connector_single_magnet (Autodesk Fusion 360 design; units mm, degrees)
Autodesk Fusion 360 part; units mm, degrees
sketch "Sketch1" plane through (0, 0, 0) normal (0, 1, 0) x (1, 0, 0)
  line L0 (0, 0) -> (-34, 0)
  line L1 (-34, 0) -> (-34, -10)
  line L2 (-34, -10) -> (0, -10)
  line L3 (0, -10) -> (0, 0)
  line L4 (0, -5) -> (-34, -5) construction
  circle A0 centre (-17, -5) radius 4
  circle A1 centre (-30, -5) radius 2
  line L5 (-17, -2.5) -> (0, -2.5) construction
  line L6 (-17, -5) -> (-17, 0) construction
  line L7 (-17, -5) -> (-17, -10) construction
  line L8 (-22, -5) -> (-27, -5)
  arc A2 (-22, -5) -> (-27, -5) centre (-24.5, -5) ccw
  arc A3 (-27, -5) -> (-22, -5) centre (-24.5, -5) ccw
  line L9 (-7, -5) -> (-12, -5)
  arc A4 (-7, -5) -> (-12, -5) centre (-9.5, -5) ccw
  arc A5 (-12, -5) -> (-7, -5) centre (-9.5, -5) ccw
  line L10 (-9.5, -5) -> (-9.5, -10) construction
  line L11 (-9.5, -5) -> (-9.5, 0) construction
  line L12 (-30, -5) -> (-30, -10) construction
  line L13 (-30, -5) -> (-30, 0) construction
  circle A6 centre (-9.5, -5) radius 3.5
  circle A7 centre (-17, -5) radius 5
  circle A8 centre (-24.5, -5) radius 3.5
  circle A9 centre (-30, -5) radius 3
  line L14 (-8.8, -1.5707) -> (-16, -0.101)
  line L15 (-8.8, -8.4293) -> (-16, -9.899)
  line L16 (-25.2, -8.4293) -> (-18, -9.899)
  line L17 (-18, -0.101) -> (-25.2, -1.5707)
  line L18 (-24.8182, -1.5145) -> (-30.2727, -2.0124)
  line L19 (-24.8182, -8.4855) -> (-30.2727, -7.9876)
  dimension "d2" = 8
  dimension "d3" = 10
  dimension "d4" = 5
  dimension "d5" = 5
  dimension "d6" = 7.5
  dimension "d7" = 7.5
  dimension "d8" = 5.5
  dimension "d9" = 4
  dimension "d12" = 4
  dimension "d41" = 6
  dimension "d42" = 7
  dimension "d43" = 10
  dimension "d44" = 7
  constraint horizontal L0
  constraint vertical L1
  constraint horizontal L2
  constraint vertical L3
  constraint coincident L0.start L3.end
  constraint midpoint L3 L4.start
  constraint midpoint L1 L4.end
  constraint midpoint L4 A0.centre
  constraint coincident L4 A4.centre
  constraint coincident L3 L5.end
  constraint perpendicular L3 L5
  constraint coincident A0.centre L6.start
  constraint midpoint L0 L6.end
  constraint midpoint L2 L7.end
  constraint midpoint L5.start L6
  constraint coincident L4 A2.centre
  constraint coincident L4 L8.start
  constraint coincident L4 L8.end
  constraint coincident A2.centre A3.centre
  constraint coincident L4 L9.start
  constraint coincident L4 L9.end
  constraint coincident A4.centre A5.centre
  constraint coincident L4 A1.centre
  constraint coincident L2 L10.end
  constraint perpendicular L2 L10
  constraint coincident L0 L11.end
  constraint perpendicular L0 L11
  constraint coincident A1.centre L12.start
  constraint coincident L2 L12.end
  constraint perpendicular L2 L12
  constraint coincident L0 L13.end
  constraint perpendicular L0 L13
  constraint concentric A4 A6
  constraint concentric A0 A7
  constraint concentric A2 A8
  constraint tangent A7 L14
  constraint tangent A6 L14
  constraint coincident A7 L14.end
  constraint coincident A6 L14.start
  constraint tangent A7 L15
  constraint tangent A6 L15
  constraint tangent A8 L16
  constraint tangent A7 L16
  constraint tangent A8 L17
  constraint tangent A7 L17
  constraint tangent A9 L18
  constraint tangent A8 L18
  constraint tangent A9 L19
  constraint tangent A8 L19
  constraint coincident A7 L15.end
  constraint coincident A6 L15.start
  constraint coincident A7 L17.start
  constraint coincident A7 L16.end
  constraint coincident A8 L16.start
  constraint coincident A8 L19.start
  constraint coincident A9 L19.end
  constraint coincident A8 L18.start
  constraint coincident A8 L17.end
  constraint coincident A9 L18.end
  measures "d2" diameter of A0
  measures "d3" distance of L0.start L2.end
  measures "d4" diameter of A4
  measures "d5" diameter of A2
  measures "d6" distance of A0.centre A4.centre
  measures "d7" distance of A0.centre A2.centre
  measures "d8" horizontal distance of A2.centre A1.centre
  measures "d9" diameter of A1
  measures "d12" distance of L1 A1.centre
  measures "d41" diameter of A9
  measures "d42" diameter of A8
  measures "d43" diameter of A7
  measures "d44" diameter of A6
extrude "Extrude1" add sketch "Sketch1" along normal blind 3 contours A0 A6 A7 A8 | A6 A7 L14 | A7 A8 L17 L18 | A0 A6 A7 A8 | A6 A7 | L9 A4 | L9 A5 | A6 A7 | A7 A8 | A2 A7 A8 A9 | A8 L17 L18 | A8 A9 L17 L18 | A7 A8 L16 L19 | A6 A7 L15 | L8 A3 | L8 A2 | A3 A7 A8 A9 | A8 A9 | A8 A9 L16 L19 | A8 L16 L19 | A8 A9
revolve "Revolve2" add sketch "Sketch1" angle 360 about axis through (0, 0, 5) along (-1, 0, 0) contours L9 A4 | L8 A2
ref_plane "WorkPlane2" through (0, 1.5, 0) normal (0, 1, 0) x (0, 0, 1)
sketch "Sketch2" plane through (0, 0, 0) normal (1, 0, 0) x (0, 1, 0)
  line L0 (0, 10) -> (-1.8, 10)
  line L1 (-1.8, 10) -> (-1.8, 0)
  line L2 (-1.8, 0) -> (0, 0)
  line L3 (0, 0) -> (0, 10)
  line L4 (-1.8, 10) -> (-10.0906, 10)
  line L5 (-10.0906, 10) -> (-10.0906, 0.2529)
  line L6 (-10.0906, 0.2529) -> (-1.8, 0.2529)
  line L7 (-1.8, 0.2529) -> (-1.8, 10)
  dimension "d25" = 1.8
  constraint horizontal L0
  constraint vertical L1
  constraint horizontal L2
  constraint vertical L3
  constraint coincident L2.end L3.start
  constraint horizontal L4
  constraint vertical L5
  constraint horizontal L6
  constraint vertical L7
  measures "d25" distance of L0.start L0.end
sketch "Sketch3" plane through (0, 3, 0) normal (0, 1, 0) x (-1, 0, 0)
  circle A0 centre (30, 5) radius 2
  circle A1 centre (9.5, 5) radius 2.4871
  circle A2 centre (24.5, 5) radius 2.5
  line L0 (25.7894, 7.1418) -> (23.2106, 7.1418)
  line L1 (11.9871, 5) -> (7.0129, 5)
  arc A3 (27, 5) -> (22, 5) centre (24.5, 5) ccw
  line L2 (27, 5) -> (22, 5)
  arc A4 (16, 0.101) -> (18, 0.101) centre (17, 5) ccw
  line L3 (18, 0.101) -> (25.0106, 1.5321)
  line L4 (25.0106, 1.5321) -> (30.2727, 2.0124)
  arc A5 (30.2727, 2.0124) -> (30.2727, 7.9876) centre (30, 5) ccw
  line L5 (30.2727, 7.9876) -> (25.0106, 8.4679)
  line L6 (25.0106, 8.4679) -> (18, 9.899)
  circle A6 centre (17, 5) radius 4
  arc A7 (8.8, 8.4293) -> (8.8, 1.5707) centre (9.5, 5) ccw
  line L7 (8.8, 1.5707) -> (16, 0.101)
  arc A8 (18, 9.899) -> (16, 9.899) centre (17, 5) ccw
  line L8 (16, 9.899) -> (8.8, 8.4293)
  dimension "d30" = 15
  dimension "d31" = 4.9742
  dimension "d32" = 5
  constraint coincident A2 L0.start
  constraint coincident A2 L0.end
  constraint horizontal L0
  constraint coincident A1 L1.start
  constraint coincident A1 L1.end
  constraint parallel L0 L1
  constraint concentric A2 A3
  constraint coincident A3.start L2.start
  constraint coincident A3.end L2.end
  measures "d30" distance of A1.centre A2.centre
  measures "d31" diameter of A1
  measures "d32" diameter of A2
revolve "Revolve3" cut sketch "Sketch3" angle 360 about axis through (-27, 3, 5) along (1, 0, 0) contours A1 L1 | A2 L2 picked at (9.562, 4.1733)
extrude "Extrude3" cut sketch "Sketch2" against normal blind 34 contours L1 L4 L5 L6 L7
extrude "Extrude4" add sketch "Sketch3" along normal blind 0.6 from surface at -2.5 contours A1 L1 | A1 L1 | A2 L0 A3 L2 | A2 L2 | A2 L0 A3
move_face "OffsetFaces2" offset -0.1 2 faces at (-7.6693, 2.6754, 6.652) (-22.6598, 2.6737, 6.6605)
ref_plane "WorkPlane3" through (0, 0, 5) normal (0, 0, 1) x (1, 0, 0)
equation "d3 = d2 + 2 mm"
equation "d5 = d4"
equation "d6 = d4 / 2 + d2 / 2 + 1 mm"
equation "d7 = d6"
equation "d8 = d5 / 2 + d9 / 2 + 1 mm"
equation "d41 = d9 + 2 mm"
equation "d42 = d5 + 2 mm"
equation "d43 = d2 + 2 mm"
equation "d44 = d4 + 2 mm"
